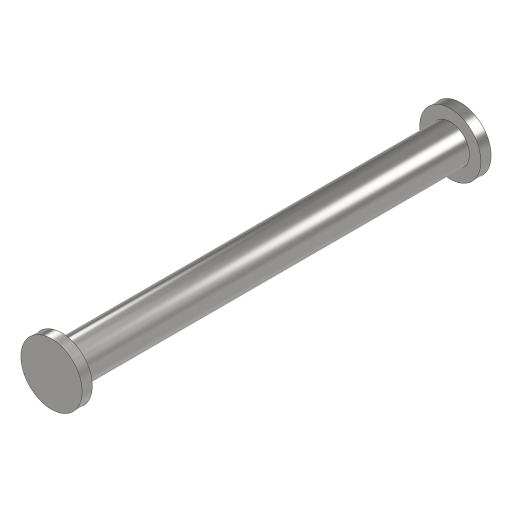
# Autodesk Inventor part: trzpien
Saved by Autodesk Inventor 2023.2 (Build 272271000, 271)
## iProperties
Created: 2022-12-05
Part Number: trzpien
Material: Stainless Steel
Document SubType Name: Modeling
Designer: GUT
Mass: 30.5504 g
Surface Area: 23.1025 cm^2
Volume: 3.8188 cm^3
Density: 8 g/cm^3
Appearance: Semi-Polished
Author: GUT
Autodesk Inventor part; units mm, degrees
ref_plane "YZ Plane" through (0, 0, 0) normal (1, 0, 0) x (0, 1, 0)
ref_plane "XZ Plane" through (0, 0, 0) normal (0, 1, 0) x (-1, 0, 0)
ref_plane "XY Plane" through (0, 0, 0) normal (0, 0, 1) x (1, 0, 0)
sketch "Sketch1" plane through (0, 0, 0) normal (1, 0, 0) x (0, 1, 0)
  line L0 (11.7841, 107.8183) -> (15.5341, 107.8183)
  line L1 (15.5341, 107.8183) -> (15.5341, 31.6183)
  line L2 (15.5341, 31.6183) -> (11.7841, 31.6183)
  line L3 (11.7841, 31.6183) -> (11.7841, 107.8183)
  line L4 (11.7841, 107.8183) -> (17.7841, 107.8183)
  line L5 (17.7841, 107.8183) -> (17.7841, 109.8183)
  line L6 (17.7841, 109.8183) -> (11.7841, 109.8183)
  line L7 (11.7841, 109.8183) -> (11.7841, 107.8183)
  line L8 (11.7841, 31.6183) -> (17.7841, 31.6183)
  line L9 (17.7841, 31.6183) -> (17.7841, 29.6183)
  line L10 (17.7841, 29.6183) -> (11.7841, 29.6183)
  line L11 (11.7841, 29.6183) -> (11.7841, 31.6183)
  point P0 (0, 0)
  point P1 (15.5341, 31.6183)
  dimension "d0" = 3.75
  dimension "d1" = 76.2
  dimension "d2" = 6
  dimension "d3" = 2
  constraints: 24 end point, 6 parallel, 3 horizontal, 3 perpendicular, 2 equal length
  measures "d0" distance of L1.end L2.end
  measures "d1" distance of L0.end L1.end
  measures "d2" distance of L6.end L5.end
  measures "d3" distance of L4.end L5.end
revolve "Revolution1" add sketch "Sketch1" angle 360 about axis through (0, 11.7841, 31.6183) along (0, 0, 1)
body "Solid1"
